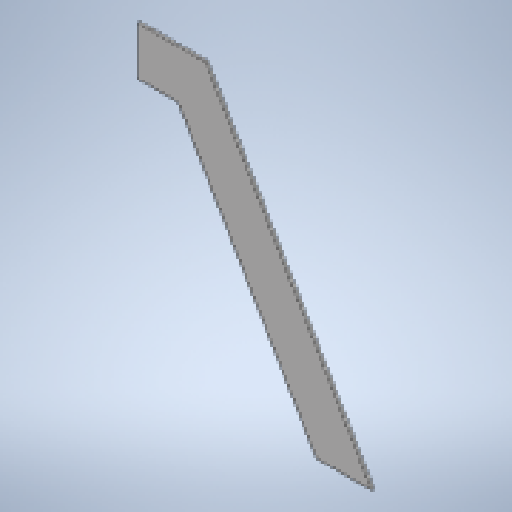
# Autodesk Inventor part: MSC 202 GRID CORNER
Saved by Autodesk Inventor 2025.1 (Build 291241020, 241B)
## iProperties
Created: 2025-01-14
Part Number: MSC 202 GRID CORNER
Material: Stainless Steel
Document SubType Name: Sheet Metal
Designer: pokla
Density: 8 g/cm^3
Sheet Metal Rule: AISI304 3mm Die 32
Appearance: Default
Author: pokla
Autodesk Inventor part; units mm, degrees
ref_plane "YZ Plane" through (0, 0, 0) normal (1, 0, 0) x (0, 1, 0)
ref_plane "XZ Plane" through (0, 0, 0) normal (0, 1, 0) x (-1, 0, 0)
ref_plane "XY Plane" through (0, 0, 0) normal (0, 0, 1) x (1, 0, 0)
sketch "Sketch1" plane through (0, 0, 0) normal (0, 1, 0) x (-1, 0, 0)
  line L0 (171.3139, 357) -> (-34.634, 0)
  line L1 (-34.634, 0) -> (34.634, 0)
  line L2 (34.634, 0) -> (205.9689, 297)
  line L3 (205.9689, 297) -> (255.9689, 297)
  line L4 (255.9689, 297) -> (255.9689, 357)
  line L5 (255.9689, 357) -> (171.3139, 357)
  point P0 (0, 0)
  point P1 (0, 0)
  dimension "d0" = 50
  dimension "d1" = 60
  dimension "d3" = 119.98
  dimension "d4" = 297
  dimension "d5" = 60
  measures "d0" distance of L2.end L3.end
  measures "d1" distance between parallel lines of L0 L2
  measures "d3" angle of L0 L5
  measures "d4" distance between parallel lines of L1 L3
  measures "d5" distance between parallel lines of L3 L5
extrude "Plate1" add sketch "Sketch1" along normal mid plane 3
equation "\"d5\" = d1"
equation "\"d6\" = Thickness"
equation "\"BendReliefWidth\" = Thickness"
equation "\"BendReliefDepth\" = 0.5 * Thickness"
equation "\"CornerReliefSize\" = 4 * Thickness"
equation "\"MinimumRemnant\" = 2 * Thickness"
equation "\"TransitionRadius\" = BendRadius"
equation "\"JacobiRadiusSize\" = BendRadius"
equation "\"GapSize\" = Thickness"
equation "\"Thickness\" = 3"
equation "\"BendRadius\" = 5"
body "Solid1"
